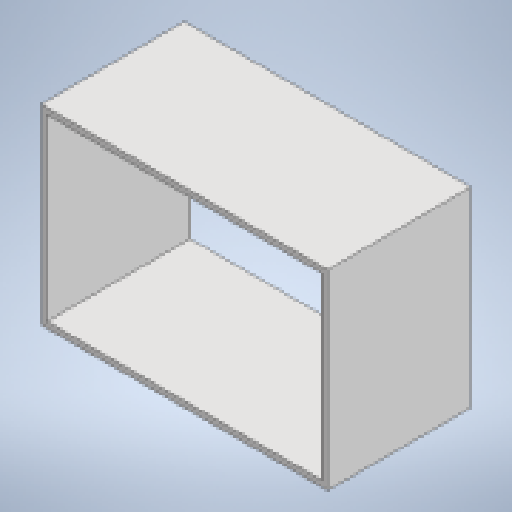
# Autodesk Inventor part: YGANTRYTUBE
Saved by Autodesk Inventor 2023 (Build 270158000, 158)
## iProperties
Created: 2022-05-03
Part Number: YGANTRYTUBE
Material: Generic
Document SubType Name: Modeling
Designer: plebbb
Density: 1 g/cm^3
Appearance: Default
Author: plebbb
Autodesk Inventor part; units mm, degrees
ref_plane "YZ Plane" through (0, 0, 0) normal (1, 0, 0) x (0, 1, 0)
ref_plane "XZ Plane" through (0, 0, 0) normal (0, 1, 0) x (-1, 0, 0)
ref_plane "XY Plane" through (0, 0, 0) normal (0, 0, 1) x (1, 0, 0)
sketch "Sketch1" plane through (0, 0, 0) normal (0, 0, 1) x (1, 0, 0)
  line L0 (0, 0) -> (152.4, 0)
  line L1 (152.4, 0) -> (152.4, 101.6)
  line L2 (152.4, 101.6) -> (0, 101.6)
  line L3 (0, 101.6) -> (0, 0)
  dimension "d0" = 152.4
  dimension "d1" = 101.6
  constraints: 8 end point, 2 parallel, 1 horizontal, 1 perpendicular
  measures "d0" distance of L1.end L2.end
  measures "d1" distance of L0.end L1.end
extrude "Extrusion1" add sketch "Sketch1" along normal blind 40.005
shell "Shell1" thickness 3.175 removed faces 2 at (50.8, 67.7333, 0) at (50.8, 67.7333, 40.005)
sketch "Sketch2" plane through (3.175, 98.425, 0) normal (0, -1, 0) x (1, 0, 0)
  circle A0 centre (118.025, 7.5025) radius 4
  circle A1 centre (28.025, 7.5025) radius 4
  line L0 (-3.175, 0) -> (-3.175, 40.005) construction
  line L1 (-3.175, 0) -> (149.225, 0) construction
  circle A2 centre (118.025, 32.5025) radius 4
  circle A3 centre (28.025, 32.5025) radius 4
  line L2 (118.025, 7.5025) -> (28.025, 7.5025) construction
  line L3 (28.025, 7.5025) -> (28.025, 32.5025)
  line L4 (28.025, 32.5025) -> (118.025, 32.5025) construction
  line L5 (118.025, 32.5025) -> (118.025, 7.5025) construction
  point P0 (73.025, 7.5025)
  point P1 (73.025, 0)
  point P2 (28.025, 20.0025)
  point P3 (-3.175, 20.0025)
  dimension "d5" = 8
  dimension "d6" = 25
  dimension "d7" = 90
  constraints: 8 end point, 4 centre point, 4 midpoint, 3 coincident, 3 equal radius, 2 parallel, 1 horizontal, 1 horizontal alignment, 1 perpendicular, 1 vertical alignment
  measures "d5" diameter of A0
  measures "d6" distance of L2.end L3.end
  measures "d7" distance of L2.start L2.end
extrude "Extrusion2" cut sketch "Sketch2" against normal up to surface (3.175 mm away)
body "Solid1"
